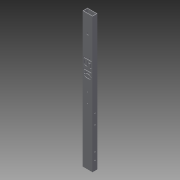
# Autodesk Inventor part: SuperSuperStructure
Saved by Autodesk Inventor 2013 (Build 170138000, 138)
## iProperties
Created: 2014-01-18
Part Number: SuperSuperStructure
Material: Generic
Document SubType Name: Modeling
Designer: 215152
Density: 1 g/cm^3
Author: 215152
Autodesk Inventor part; units mm, degrees
ref_plane "YZ Plane" through (0, 0, 0) normal (1, 0, 0) x (0, 1, 0)
ref_plane "XZ Plane" through (0, 0, 0) normal (0, 1, 0) x (-1, 0, 0)
ref_plane "XY Plane" through (0, 0, 0) normal (0, 0, 1) x (1, 0, 0)
sketch "Sketch1" plane through (0, 0, 0) normal (0, 1, 0) x (-1, 0, 0)
  line L0 (-25.4, -12.7) -> (25.4, -12.7)
  line L1 (25.4, -12.7) -> (25.4, 12.7)
  line L2 (25.4, 12.7) -> (-25.4, 12.7)
  line L3 (-25.4, 12.7) -> (-25.4, -12.7)
  line L4 (-25.4, -12.7) -> (25.4, 12.7) construction
  line L5 (25.4, -12.7) -> (-25.4, 12.7) construction
  line L6 (22.225, -9.525) -> (-22.225, -9.525)
  line L7 (-22.225, -9.525) -> (-22.225, 9.525)
  line L8 (-22.225, 9.525) -> (22.225, 9.525)
  line L9 (22.225, 9.525) -> (22.225, -9.525)
  line L10 (22.225, -9.525) -> (-22.225, 9.525) construction
  line L11 (-22.225, -9.525) -> (22.225, 9.525) construction
  point P0 (0, 0)
  dimension "d0" = 50.8
  dimension "d1" = 25.4
  dimension "d2" = 44.45
  dimension "d3" = 19.05
  constraints: 24 end point, 4 midpoint, 4 parallel, 2 horizontal, 2 perpendicular
  measures "d0" distance of L2.end L1.end
  measures "d1" distance of L1.end L0.end
  measures "d2" distance of L7.end L8.end
  measures "d3" distance of L6.end L7.end
extrude "Extrusion1" add sketch "Sketch1" along normal blind 609.6
sketch "Sketch2" plane through (-25.4, 0, 12.7) normal (0, 0, 1) x (1, 0, 0)
  line L0 (0, 609.6) -> (25.4, 609.6)
  line L1 (25.4, 609.6) -> (25.4, 584.2)
  line L2 (25.4, 584.2) -> (0, 584.2)
  line L3 (0, 584.2) -> (0, 609.6)
  circle A0 centre (25.4, 584.2) radius 6.35
  point P0 (25.4, 0)
  dimension "d6" = 25.4
  dimension "d7" = 25.4
  dimension "d8" = 12.7
  constraints: 8 end point, 2 parallel, 1 centre point, 1 coincident, 1 horizontal, 1 perpendicular
  measures "d6" distance of L1.end L2.end
  measures "d7" distance of L0.end L1.end
  measures "d8" diameter of A0
extrude "Extrusion2" cut sketch "Sketch2" against normal blind 609.6 contours A0 L2 L1 | L1 L2 A0
sketch "Sketch4" plane through (0, 0, 0) normal (0, -1, 0) x (1, 0, 0)
  line L0 (22.225, 9.525) -> (22.225, -9.525) projected
  line L1 (22.225, -9.525) -> (-22.225, -9.525) projected
  line L2 (-22.225, -9.525) -> (-22.225, 9.525) projected
  line L3 (-22.225, 9.525) -> (22.225, 9.525) projected
  line L4 (25.4, -12.7) -> (-25.4, -12.7) projected
  line L5 (25.4, 12.7) -> (25.4, -12.7) projected
  line L6 (-25.4, 12.7) -> (25.4, 12.7) projected
  line L7 (-25.4, -12.7) -> (-25.4, 12.7) projected
  point P0 (0, 0)
extrude "Extrusion4" add sketch "Sketch4" along normal blind 12.7
sketch "Sketch6" plane through (0, 609.6, 0) normal (0, 1, 0) x (1, 0, 0)
  line L0 (22.225, 9.525) -> (22.225, -9.525) projected
  line L1 (22.225, -9.525) -> (-22.225, -9.525) projected
  line L2 (-22.225, -9.525) -> (-22.225, 9.525) projected
  line L3 (-22.225, 9.525) -> (22.225, 9.525) projected
  line L4 (25.4, 12.7) -> (-25.4, 12.7) projected
  line L5 (-25.4, 12.7) -> (-25.4, -12.7) projected
  line L6 (-25.4, -12.7) -> (25.4, -12.7) projected
  line L7 (25.4, -12.7) -> (25.4, 12.7) projected
  point P0 (0, 0)
extrude "Extrusion6" add sketch "Sketch6" along normal blind 63.5
sketch "Sketch8" plane through (-25.4, -12.7, 12.7) normal (0, 0, 1) x (1, 0, 0)
  line L0 (50.8, 0) -> (50.8, 685.8) projected
  line L1 (0, 685.8) -> (50.8, 685.8) projected
  line L2 (25.4, 685.8) -> (25.4, 341.8078)
  line L3 (25.4, 685.8) -> (369.3922, 685.8) construction
  line L4 (25.4, 341.8078) -> (25.4, 291.0078)
  circle A0 centre (25.4, 291.0078) radius 3.175
  circle A1 centre (25.4, 341.8078) radius 3.175
  point P0 (25.4, 12.7)
  dimension "d49" = 343.9922
  dimension "d50" = 90
  dimension "d51" = 50.8
  dimension "d52" = 180
  dimension "d53" = 6.35
  dimension "d54" = 6.35
  constraints: 6 end point, 2 centre point, 2 coincident, 2 parallel, 1 horizontal, 1 midpoint, 1 perpendicular
  measures "d49" distance of L2.start L2.end
  measures "d50" angle of L2 L3
  measures "d51" distance of L2.end L4.end
  measures "d52" angle of L4 L2
  measures "d53" diameter of A0
  measures "d54" diameter of A1
extrude "Extrusion9" cut sketch "Sketch8" against normal blind 50.8
sketch "Sketch9" plane through (25.4, -12.7, 12.7) normal (1, 0, 0) x (0, 0, -1)
  line L0 (25.4, 0) -> (0, 0) projected
  line L1 (12.7, 0) -> (12.7, 84.1502)
  line L2 (12.7, 84.1502) -> (12.7, 46.0502)
  line L3 (12.7, 84.1502) -> (50.8, 84.1502) construction
  point P0 (12.7, 12.7)
  dimension "d57" = 84.1502
  dimension "d58" = 38.1
  dimension "d59" = 90
  constraints: 6 end point, 2 coincident, 2 perpendicular, 1 collinear, 1 horizontal, 1 midpoint
  measures "d57" distance of L1.start L1.end
  measures "d58" distance of L1.end L2.end
  measures "d59" angle of L2 L3
hole "Hole1" at (25.4, 71.4502, 0) at (25.4, 33.3502, 0) direction (-1, 0, 0) diameter 6.35 end through all
sketch "Sketch10" plane through (-25.4, -12.7, 12.7) normal (0, 0, 1) x (1, 0, 0)
  circle A0 centre (25.4, 341.8078) radius 3.175 projected
  circle A1 centre (25.4, 596.9) radius 6.35 projected
  line L0 (50.8, 0) -> (50.8, 685.8) projected
  line L1 (0, 0) -> (0, 685.8) projected
  line L2 (50.8, 0) -> (0, 0) projected
  line L3 (25.4, 341.8078) -> (25.4, 354.5078)
  line L4 (25.4, 341.8078) -> (38.1, 341.8078) construction
  line L5 (25.4, 354.5078) -> (50.8, 354.5078)
  line L6 (25.4, 354.5078) -> (0, 354.5078)
  line L7 (25.4, 596.9) -> (25.4, 501.65)
  line L8 (25.4, 501.65) -> (50.8, 501.65)
  line L9 (50.8, 501.65) -> (0, 501.65)
  line L10 (50.8, 501.65) -> (0, 501.65)
  line L11 (0, 501.65) -> (0, 354.5078)
  line L12 (0, 354.5078) -> (50.8, 354.5078)
  line L13 (50.8, 354.5078) -> (50.8, 501.65)
  line L14 (50.8, 501.65) -> (44.45, 501.65)
  line L15 (50.8, 495.3) -> (50.8, 501.65)
  line L16 (44.45, 482.6) -> (6.35, 482.6)
  line L17 (6.35, 482.6) -> (6.35, 488.95)
  line L18 (44.45, 488.95) -> (33.4515, 495.3)
  line L19 (44.45, 488.95) -> (57.15, 488.95) construction
  line L20 (33.4515, 495.3) -> (33.4515, 488.95)
  line L21 (44.45, 476.25) -> (38.1, 476.25)
  line L22 (38.1, 450.85) -> (44.45, 450.85)
  line L23 (44.45, 476.25) -> (22.225, 476.25)
  line L24 (22.225, 476.25) -> (22.225, 469.9)
  line L25 (44.45, 469.9) -> (44.45, 476.25)
  line L26 (6.35, 469.9) -> (6.35, 476.25)
  line L27 (22.225, 476.25) -> (22.225, 469.9)
  line L28 (6.35, 476.25) -> (12.7, 476.25)
  line L29 (6.35, 469.9) -> (6.35, 476.25)
  line L30 (22.225, 476.25) -> (28.575, 476.25)
  line L31 (12.7, 476.25) -> (6.35, 476.25)
  arc A2 (17.4625, 450.85) -> (28.575, 461.9625) centre (17.3488, 462.0762) ccw
  line L32 (17.4625, 450.85) -> (28.575, 461.9625) construction
  line L33 (17.4625, 450.85) -> (33.1779, 450.85) construction
  arc A3 (6.35, 461.9625) -> (17.4625, 450.85) centre (17.5762, 462.0762) ccw
  line L34 (17.4625, 450.85) -> (6.35, 461.9625) construction
  line L35 (17.4625, 450.85) -> (33.1779, 450.85) construction
  arc A4 (12.7, 461.9625) -> (22.225, 461.9625) centre (17.4625, 461.9625) ccw
  line L36 (44.45, 438.15) -> (44.45, 431.8)
  line L37 (44.45, 431.8) -> (6.35, 431.8)
  line L38 (6.35, 431.8) -> (6.35, 438.15)
  line L39 (44.45, 438.15) -> (33.4515, 444.5)
  line L40 (44.45, 438.15) -> (57.15, 438.15) construction
  line L41 (33.4515, 444.5) -> (33.4515, 438.15)
  line L42 (44.45, 431.8) -> (6.35, 431.8)
  line L43 (44.45, 412.75) -> (31.75, 425.45) construction
  line L44 (44.45, 412.75) -> (62.4105, 412.75) construction
  line L45 (44.45, 412.75) -> (31.75, 400.05) construction
  line L46 (44.45, 412.75) -> (62.4105, 412.75) construction
  line L47 (6.35, 412.75) -> (19.05, 400.05) construction
  line L48 (6.35, 412.75) -> (24.3105, 412.75) construction
  line L49 (6.35, 412.75) -> (19.05, 425.45) construction
  line L50 (6.35, 412.75) -> (24.3105, 412.75) construction
  line L51 (25.4, 425.45) -> (31.75, 425.45) construction
  line L52 (19.05, 419.1) -> (31.75, 419.1)
  line L53 (31.75, 406.4) -> (19.05, 406.4)
  line L54 (19.05, 419.1) -> (31.75, 406.4) construction
  line L55 (31.75, 419.1) -> (19.05, 406.4) construction
  line L56 (12.7, 412.75) -> (6.35, 412.75)
  line L57 (6.3002, 413.5438) -> (12.7498, 413.5438)
  line L58 (12.7498, 411.9563) -> (6.3002, 411.9563)
  line L59 (6.3002, 413.5438) -> (12.7498, 411.9563) construction
  line L60 (12.7498, 413.5438) -> (6.3002, 411.9563) construction
  line L61 (44.4998, 413.5438) -> (38.0502, 413.5438)
  line L62 (38.0502, 411.9563) -> (44.4998, 411.9563)
  line L63 (44.4998, 413.5438) -> (38.0502, 411.9563) construction
  line L64 (38.0502, 413.5438) -> (44.4998, 411.9563) construction
  line L65 (44.45, 488.95) -> (44.45, 482.6)
  line L66 (44.45, 482.6) -> (6.35, 482.6)
  line L67 (6.35, 482.6) -> (6.35, 488.95)
  line L68 (6.35, 488.95) -> (33.4515, 488.95)
  line L69 (33.4515, 488.95) -> (33.4515, 495.3)
  line L70 (33.4515, 495.3) -> (44.45, 488.95)
  line L71 (44.45, 450.85) -> (38.1, 450.85)
  line L72 (38.1, 450.85) -> (38.1, 469.9)
  line L73 (38.1, 469.9) -> (28.575, 469.9)
  line L74 (28.575, 469.9) -> (28.575, 461.9625)
  line L75 (12.7, 461.9625) -> (12.7, 476.25)
  line L76 (12.7, 476.25) -> (6.35, 476.25)
  line L77 (6.35, 476.25) -> (6.35, 461.9625)
  line L78 (22.225, 461.9625) -> (22.225, 476.25)
  line L79 (22.225, 476.25) -> (44.45, 476.25)
  line L80 (44.45, 476.25) -> (44.45, 450.85)
  line L81 (44.45, 438.15) -> (33.4515, 444.5)
  line L82 (33.4515, 444.5) -> (33.4515, 438.15)
  line L83 (33.4515, 438.15) -> (6.35, 438.15)
  line L84 (6.35, 438.15) -> (6.35, 431.8)
  line L85 (6.35, 431.8) -> (44.45, 431.8)
  line L86 (44.45, 431.8) -> (44.45, 438.15)
  line L87 (31.75, 425.45) -> (19.05, 425.45)
  line L88 (19.05, 400.05) -> (31.75, 400.05)
  line L89 (31.75, 406.4) -> (19.05, 406.4)
  line L90 (19.05, 419.1) -> (31.75, 419.1)
  arc A5 (38.0502, 413.5438) -> (31.75, 419.1) centre (31.75, 412.75) ccw
  arc A6 (31.75, 406.4) -> (38.0502, 411.9563) centre (31.75, 412.75) ccw
  arc A7 (19.05, 419.1) -> (12.7498, 413.5438) centre (19.05, 412.75) ccw
  arc A8 (12.7498, 411.9563) -> (19.05, 406.4) centre (19.05, 412.75) ccw
  arc A9 (44.4998, 413.5438) -> (31.75, 425.45) centre (31.8246, 412.7502) ccw
  arc A10 (31.75, 400.05) -> (44.4998, 411.9563) centre (31.8246, 412.7498) ccw
  arc A11 (19.05, 425.45) -> (6.3002, 413.5438) centre (18.9754, 412.7502) ccw
  arc A12 (6.3002, 411.9563) -> (19.05, 400.05) centre (18.9754, 412.7498) ccw
  point P0 (25.4, 12.7)
  point P1 (25.4, 412.75)
  point P2 (9.525, 412.75)
  point P3 (41.275, 412.75)
  dimension "d67" = 12.7
  dimension "d68" = 90
  dimension "d69" = 95.25
  dimension "d75" = 6.35
  dimension "d76" = 150
  dimension "d77" = 6.35
  dimension "d78" = 6.35
  dimension "d79" = 25.4
  dimension "d80" = 22.225
  dimension "d81" = 6.35
  dimension "d82" = 15.875
  dimension "d83" = 6.35
  dimension "d87" = 45
  dimension "d88" = 11.2268
  dimension "d89" = 135
  dimension "d90" = 11.2268
  dimension "d95" = 38.1
  dimension "d96" = 6.35
  dimension "d97" = 12.7
  dimension "d98" = 150
  dimension "d103" = 135
  dimension "d105" = 135
  dimension "d107" = 45
  dimension "d109" = 45
  dimension "d114" = 12.7
  dimension "d115" = 12.7
  dimension "d118" = 1.5875
  dimension "d119" = 6.35
  dimension "d120" = 6.35
  dimension "d121" = 6.35
  dimension "d122" = 6.35
  dimension "d123" = 12.7
  dimension "d124" = 12.7
  dimension "d125" = 12.7
  dimension "d126" = 12.7
  dimension "d127" = 12.7
  dimension "d128" = 6.35
  dimension "d129" = 25.4
  constraints: 176 end point, 22 point on circle, 19 horizontal, 19 perpendicular, 11 centre point, 11 parallel, 9 equal length, 7 midpoint, 5 collinear, 4 point on line, 2 tangent
  measures "d67" distance of L3.start L3.end
  measures "d68" angle of L4 L3
  measures "d69" distance of L7.start L7.end
  measures "d75" distance of L16.end L17.end
  measures "d76" angle of L19 L18
  measures "d77" distance of L16.start L21.start
  measures "d78" distance of L21.start L21.end
  measures "d79" distance of L21.end L22.start
  measures "d80" distance of L25.start L24.end
  measures "d81" distance of L24.end L23.end
  measures "d82" distance of L26.end L27.start
  measures "d83" distance of L26.start L26.end
  measures "d87" angle of L33 L32
  measures "d88" radius of A2
  measures "d89" angle of L35 L34
  measures "d90" radius of A3
  measures "d95" distance of L36.end L37.end
  measures "d96" distance of L36.start L36.end
  measures "d97" distance of L36.start L39.end
  measures "d98" angle of L40 L39
  measures "d103" angle of L44 L43
  measures "d105" angle of L45 L46
  measures "d107" angle of L47 L48
  measures "d109" angle of L50 L49
  measures "d114" distance of L53.start L53.end
  measures "d115" distance of L52.end L53.start
  measures "d118" distance of L57.end L58.start
  measures "d119" radius of A5
  measures "d120" radius of A6
  measures "d121" radius of A7
  measures "d122" radius of A8
  measures "d123" radius of A9
  measures "d124" radius of A10
  measures "d125" radius of A11
  measures "d126" radius of A12
  measures "d127" distance between parallel lines of L22 L83
  measures "d128" distance of L39.end L41.end
  measures "d129" distance between parallel lines of L22 L23
extrude "Extrusion10" cut sketch "Sketch10" against normal blind 6.35 contours L16 L17 L68 L20 L18 L65 | L25 L80 L22 L72 L73 L74 A2 A3 L77 L26 L28 L75 A4 L78 L24 L23 L21 | L36 L37 L38 L83 L41 L39 | A7 L57 A11 L87 A9 L61 A5 L52 | A6 L62 A10 L88 A12 L58 A8 L53
sketch "Sketch11" plane through (25.4, -12.7, 12.7) normal (1, 0, 0) x (0, 0, -1)
  line L0 (0, 685.8) -> (25.4, 685.8) projected
  line L1 (0, 0) -> (0, 685.8) projected
  line L2 (12.7, 685.8) -> (12.7, 254)
  line L3 (12.7, 685.8) -> (444.5, 685.8) construction
  line L4 (12.7, 254) -> (12.7, 203.2)
  circle A0 centre (12.7, 254) radius 3.175
  circle A1 centre (12.7, 203.2) radius 3.175
  point P0 (12.7, 12.7)
  dimension "d132" = 431.8
  dimension "d133" = 90
  dimension "d134" = 50.8
  dimension "d135" = 180
  dimension "d136" = 6.35
  dimension "d137" = 6.35
  constraints: 6 end point, 2 centre point, 2 coincident, 2 parallel, 1 horizontal, 1 midpoint, 1 perpendicular
  measures "d132" distance of L2.start L2.end
  measures "d133" angle of L2 L3
  measures "d134" distance of L2.end L4.end
  measures "d135" angle of L4 L2
  measures "d136" diameter of A0
  measures "d137" diameter of A1
extrude "Extrusion11" cut sketch "Sketch11" against normal blind 50.8
body "Solid1"
